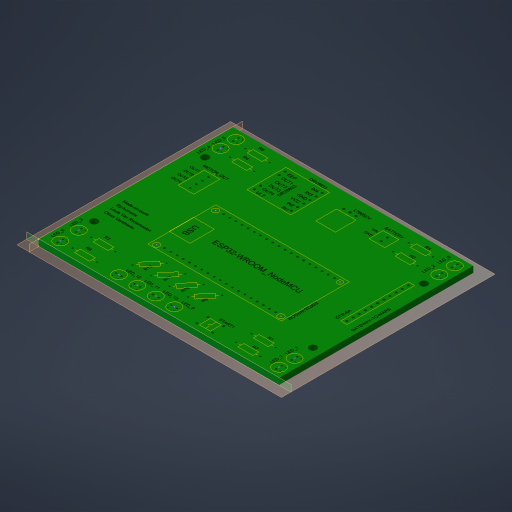
# Autodesk Inventor part: PCB
Saved by Autodesk Inventor 2024 (Build 280153000, 153)
## iProperties
Manager: Louis Van Roosmaelen
Company: DCS - DIGITAL COMBAT SIMULATOR
Created: 2023-12-13
Part Number: PCB
Material: S235
Catalog Web Link: http://emmausbovenbouw.op-weg.be/
Vendor: Emmaüsinstituut Bovenbouw Aalter
Document SubType Name: Modeling
Designer: Louis
Engineer: Declercq St.
Manufacturer: Standard
Standards Organization: Custom
Density: 7.86 g/cm^3
Appearance: Steel
IDENT.NR.: AJ2022
TEAM: 30
Title: F18C Home Cockpit
Author: Louis
Keywords: Ø
Autodesk Inventor part; units mm, degrees
sketch "Outline" plane through (0, 0, 0) normal (0, 0, 1) x (1, 0, 0)
  line L0 (0, 80) -> (99.0602, 80.0102)
  line L1 (99.0602, 80.0102) -> (99.0602, 0)
  line L2 (99.0602, 0) -> (0, 0)
  line L3 (0, 0) -> (0, 80)
  constraints: 8 end point
extrude "Extrusion2" add sketch "Outline" along normal blind 2.5
sketch "Sketch3" plane through (0, 0, 2.5) normal (0, 0, 1) x (1, 0, 0)
  circle A0 centre (71.3201, 72.3901) radius 0.5169
  circle A1 centre (71.32, 72.3901) radius 0.7754
  circle A2 centre (92.7102, 44.4501) radius 0.5159
  circle A3 centre (5.08, 75.0601) radius 0.4226
  circle A4 centre (71.3201, 69.8501) radius 0.5169
  circle A5 centre (71.32, 69.8501) radius 0.7754
  circle A6 centre (5.08, 75.0602) radius 0.9508
  circle A7 centre (92.7102, 44.4501) radius 0.8254
  circle A8 centre (12.9, 57.15) radius 0.4369
  circle A9 centre (12.8999, 57.1499) radius 0.6554
  circle A10 centre (87.5502, 68.5801) radius 0.3637
  circle A11 centre (5.08, 77.3402) radius 0.4226
  circle A12 centre (12.9, 54.61) radius 0.4369
  circle A13 centre (12.8999, 54.6099) radius 0.6554
  circle A14 centre (5.08, 77.3404) radius 0.9508
  circle A15 centre (87.5502, 68.5801) radius 0.6754
  circle A16 centre (12.9, 52.07) radius 0.4369
  circle A17 centre (12.8999, 52.0699) radius 0.6554
  circle A18 centre (92.7102, 41.9101) radius 0.5159
  circle A19 centre (50.93, 3.81) radius 0.4226
  circle A20 centre (12.9, 49.53) radius 0.4369
  circle A21 centre (12.8999, 49.5298) radius 0.6554
  circle A22 centre (50.9301, 3.81) radius 0.9508
  circle A23 centre (92.7102, 41.9101) radius 0.8254
  circle A24 centre (26.6701, 62.2301) radius 0.544
  circle A25 centre (26.6701, 62.2301) radius 0.8
  circle A26 centre (10.24, 68.5801) radius 0.3637
  circle A27 centre (53.2101, 3.81) radius 0.4226
  circle A28 centre (26.6701, 64.7701) radius 0.544
  circle A29 centre (26.6701, 64.7701) radius 0.8
  circle A30 centre (53.2103, 3.81) radius 0.9508
  circle A31 centre (10.24, 68.5801) radius 0.6754
  circle A32 centre (26.6701, 67.3101) radius 0.544
  circle A33 centre (26.6701, 67.3101) radius 0.8
  circle A34 centre (92.7102, 39.3701) radius 0.5159
  circle A35 centre (43.31, 3.81) radius 0.4226
  circle A36 centre (26.6701, 69.8501) radius 0.544
  circle A37 centre (26.6701, 69.8501) radius 0.8
  circle A38 centre (43.3101, 3.81) radius 0.9508
  circle A39 centre (92.7102, 39.3701) radius 0.8254
  circle A40 centre (26.6701, 72.3901) radius 0.544
  circle A41 centre (26.6701, 72.3901) radius 0.8
  circle A42 centre (20.24, 11.43) radius 0.3637
  circle A43 centre (45.5901, 3.81) radius 0.4226
  circle A44 centre (26.6701, 74.9301) radius 0.544
  circle A45 centre (26.6701, 74.9301) radius 0.8
  circle A46 centre (45.5903, 3.81) radius 0.9508
  circle A47 centre (20.24, 11.43) radius 0.6754
  circle A48 centre (41.9101, 62.2301) radius 0.544
  circle A49 centre (41.9101, 62.2301) radius 0.8
  circle A50 centre (92.7102, 36.8301) radius 0.5159
  circle A51 centre (35.69, 3.81) radius 0.4226
  circle A52 centre (41.9101, 64.7701) radius 0.544
  circle A53 centre (41.9101, 64.7701) radius 0.8
  circle A54 centre (35.6901, 3.81) radius 0.9508
  circle A55 centre (92.7102, 36.8301) radius 0.8254
  circle A56 centre (41.9101, 67.3101) radius 0.544
  circle A57 centre (41.9101, 67.3101) radius 0.8
  circle A58 centre (87.5502, 74.9301) radius 0.3637
  circle A59 centre (37.9701, 3.81) radius 0.4226
  circle A60 centre (41.9101, 69.8501) radius 0.544
  circle A61 centre (41.9101, 69.8501) radius 0.8
  circle A62 centre (37.9703, 3.81) radius 0.9508
  circle A63 centre (87.5502, 74.9301) radius 0.6754
  circle A64 centre (41.9101, 72.3901) radius 0.544
  circle A65 centre (41.9101, 72.3901) radius 0.8
  circle A66 centre (92.7102, 34.2901) radius 0.5159
  circle A67 centre (28.07, 3.81) radius 0.4226
  circle A68 centre (41.9101, 74.9301) radius 0.544
  circle A69 centre (41.9101, 74.9301) radius 0.8
  circle A70 centre (28.0701, 3.81) radius 0.9508
  circle A71 centre (92.7102, 34.2901) radius 0.8254
  circle A72 centre (95.2502, 9.0199) radius 0.4226
  circle A73 centre (95.2502, 9.0201) radius 0.9508
  circle A74 centre (10.24, 11.43) radius 0.3637
  circle A75 centre (30.3501, 3.81) radius 0.4226
  circle A76 centre (95.2502, 11.3001) radius 0.4226
  circle A77 centre (95.2502, 11.3002) radius 0.9508
  circle A78 centre (30.3503, 3.81) radius 0.9508
  circle A79 centre (10.24, 11.43) radius 0.6754
  circle A80 centre (95.2502, 68.7101) radius 0.4226
  circle A81 centre (95.2502, 68.7102) radius 0.9508
  circle A82 centre (77.5502, 10.16) radius 0.3637
  circle A83 centre (92.7102, 59.6901) radius 0.5159
  circle A84 centre (95.2502, 70.9902) radius 0.4226
  circle A85 centre (95.2502, 70.9903) radius 0.9508
  circle A86 centre (77.5502, 10.16) radius 0.6754
  circle A87 centre (92.7102, 57.1501) radius 0.5159
  circle A88 centre (5.08, 10.2899) radius 0.4226
  circle A89 centre (5.08, 10.2901) radius 0.9508
  circle A90 centre (92.7102, 57.1501) radius 0.8254
  circle A91 centre (77.5502, 74.9301) radius 0.3637
  circle A92 centre (5.08, 12.5701) radius 0.4226
  circle A93 centre (5.08, 12.5702) radius 0.9508
  circle A94 centre (77.5502, 74.9301) radius 0.6754
  circle A95 centre (92.7102, 54.6101) radius 0.5159
  circle A96 centre (5.08, 68.7101) radius 0.4226
  circle A97 centre (5.08, 68.7102) radius 0.9508
  circle A98 centre (92.7102, 54.6101) radius 0.8254
  circle A99 centre (87.5502, 10.16) radius 0.3637
  circle A100 centre (5.08, 70.9902) radius 0.4226
  circle A101 centre (5.08, 70.9903) radius 0.9508
  circle A102 centre (87.5502, 10.16) radius 0.6754
  circle A103 centre (92.7102, 52.0701) radius 0.5159
  circle A104 centre (95.2502, 75.0601) radius 0.4226
  circle A105 centre (95.2502, 75.0602) radius 0.9508
  circle A106 centre (92.7102, 52.0701) radius 0.8254
  circle A107 centre (20.24, 68.5801) radius 0.3637
  circle A108 centre (95.2502, 77.3402) radius 0.4226
  circle A109 centre (95.2502, 77.3404) radius 0.9508
  circle A110 centre (20.24, 68.5801) radius 0.6754
  circle A111 centre (92.7102, 49.5301) radius 0.5159
  circle A112 centre (5.08, 2.6699) radius 0.4226
  circle A113 centre (5.08, 2.6701) radius 0.9508
  circle A114 centre (92.7102, 49.5301) radius 0.8254
  circle A115 centre (77.5502, 68.5801) radius 0.3637
  circle A116 centre (5.08, 4.95) radius 0.4226
  circle A117 centre (5.08, 4.9502) radius 0.9508
  circle A118 centre (77.5502, 68.5801) radius 0.6754
  circle A119 centre (92.7102, 46.9901) radius 0.5159
  circle A120 centre (95.2502, 2.6699) radius 0.4226
  circle A121 centre (95.2502, 2.6701) radius 0.9508
  circle A122 centre (92.7102, 46.9901) radius 0.8254
  circle A123 centre (20.24, 3.81) radius 0.3637
  circle A124 centre (95.2502, 4.95) radius 0.4226
  circle A125 centre (95.2502, 4.9502) radius 0.9508
  circle A126 centre (20.24, 3.81) radius 0.6754
  circle A127 centre (10.24, 3.81) radius 0.3637
  circle A128 centre (10.24, 3.81) radius 0.6754
  circle A129 centre (77.5502, 3.81) radius 0.3637
  circle A130 centre (77.5502, 3.81) radius 0.6754
  circle A131 centre (87.5502, 3.81) radius 0.3637
  circle A132 centre (87.5502, 3.81) radius 0.6754
  circle A133 centre (20.24, 74.9301) radius 0.3637
  circle A134 centre (20.24, 74.9301) radius 0.6754
  circle A135 centre (10.24, 74.9301) radius 0.3637
  circle A136 centre (10.24, 74.9301) radius 0.6754
  circle A137 centre (57.8241, 17.8003) radius 0.3637
  circle A138 centre (57.824, 17.8004) radius 0.6754
  circle A139 centre (51.3962, 10.1398) radius 0.3637
  circle A140 centre (51.3962, 10.1397) radius 0.6754
  circle A141 centre (50.204, 17.8002) radius 0.3637
  circle A142 centre (50.204, 17.8004) radius 0.6754
  circle A143 centre (43.7762, 10.1398) radius 0.3637
  circle A144 centre (43.7762, 10.1397) radius 0.6754
  circle A145 centre (42.584, 17.8003) radius 0.3637
  circle A146 centre (42.5839, 17.8004) radius 0.6754
  circle A147 centre (36.1561, 10.1398) radius 0.3637
  circle A148 centre (36.1562, 10.1397) radius 0.6754
  circle A149 centre (34.964, 17.8003) radius 0.3637
  circle A150 centre (34.9639, 17.8004) radius 0.6754
  circle A151 centre (28.5361, 10.1398) radius 0.3637
  circle A152 centre (28.5362, 10.1397) radius 0.6754
  circle A153 centre (62.6802, 2.54) radius 0.5167
  circle A154 centre (62.6802, 2.54) radius 0.7874
  circle A155 centre (69.1801, 2.54) radius 0.5167
  circle A156 centre (69.1801, 2.54) radius 0.7874
  circle A157 centre (69.1801, 7.0399) radius 0.5167
  circle A158 centre (69.1801, 7.0399) radius 0.7874
  circle A159 centre (62.6802, 7.0399) radius 0.5167
  circle A160 centre (62.6802, 7.0399) radius 0.7874
  circle A161 centre (52.0701, 73.6601) radius 0.5672
  circle A162 centre (54.6101, 73.6601) radius 0.5672
  circle A163 centre (54.6101, 73.6601) radius 0.825
  circle A164 centre (57.1501, 73.6601) radius 0.5672
  circle A165 centre (57.1501, 73.6601) radius 0.825
  circle A166 centre (74.9301, 22.733) radius 0.4877
  circle A167 centre (74.9301, 22.733) radius 0.8128
  circle A168 centre (72.3901, 22.733) radius 0.4877
  circle A169 centre (72.3901, 22.733) radius 0.8128
  circle A170 centre (69.8501, 22.733) radius 0.4877
  circle A171 centre (69.8501, 22.733) radius 0.8128
  circle A172 centre (67.3101, 22.733) radius 0.4877
  circle A173 centre (67.3101, 22.733) radius 0.8128
  circle A174 centre (64.7701, 22.733) radius 0.4877
  circle A175 centre (64.7701, 22.733) radius 0.8128
  circle A176 centre (62.2301, 22.733) radius 0.4877
  circle A177 centre (62.2301, 22.733) radius 0.8128
  circle A178 centre (59.6901, 22.733) radius 0.4877
  circle A179 centre (59.6901, 22.733) radius 0.8128
  circle A180 centre (57.1501, 22.733) radius 0.4877
  circle A181 centre (57.1501, 22.733) radius 0.8128
  circle A182 centre (54.6101, 22.733) radius 0.4877
  circle A183 centre (54.6101, 22.733) radius 0.8128
  circle A184 centre (52.0701, 22.733) radius 0.4877
  circle A185 centre (52.0701, 22.733) radius 0.8128
  circle A186 centre (49.5301, 22.733) radius 0.4877
  circle A187 centre (49.5301, 22.733) radius 0.8128
  circle A188 centre (46.9901, 22.733) radius 0.4877
  circle A189 centre (46.9901, 22.733) radius 0.8128
  circle A190 centre (44.4501, 22.733) radius 0.4877
  circle A191 centre (44.4501, 22.733) radius 0.8128
  circle A192 centre (41.9101, 22.733) radius 0.4877
  circle A193 centre (41.9101, 22.733) radius 0.8128
  circle A194 centre (39.3701, 22.733) radius 0.4877
  circle A195 centre (39.3701, 22.733) radius 0.8128
  circle A196 centre (36.8301, 22.733) radius 0.4877
  circle A197 centre (36.8301, 22.733) radius 0.8128
  circle A198 centre (34.2901, 22.733) radius 0.4877
  circle A199 centre (34.2901, 22.733) radius 0.8128
  circle A200 centre (31.7501, 22.733) radius 0.4877
  circle A201 centre (31.7501, 22.733) radius 0.8128
  circle A202 centre (29.0831, 22.733) radius 0.4877
  circle A203 centre (29.0831, 22.733) radius 0.8128
  circle A204 centre (29.151, 47.0041) radius 0.4877
  circle A205 centre (29.1509, 47.0041) radius 0.8128
  circle A206 centre (31.691, 47.0041) radius 0.4877
  circle A207 centre (31.6909, 47.0041) radius 0.8128
  circle A208 centre (34.231, 47.0041) radius 0.4877
  circle A209 centre (34.2309, 47.0041) radius 0.8128
  circle A210 centre (36.771, 47.0041) radius 0.4877
  circle A211 centre (36.7709, 47.0041) radius 0.8128
  circle A212 centre (39.311, 47.0041) radius 0.4877
  circle A213 centre (39.3109, 47.0041) radius 0.8128
  circle A214 centre (41.851, 47.0041) radius 0.4877
  circle A215 centre (41.8509, 47.0041) radius 0.8128
  circle A216 centre (44.391, 47.0041) radius 0.4877
  circle A217 centre (44.3909, 47.0041) radius 0.8128
  circle A218 centre (46.931, 47.0041) radius 0.4877
  circle A219 centre (46.9309, 47.0041) radius 0.8128
  circle A220 centre (49.471, 47.0041) radius 0.4877
  circle A221 centre (49.4709, 47.0041) radius 0.8128
  circle A222 centre (52.011, 47.0041) radius 0.4877
  circle A223 centre (52.0109, 47.0041) radius 0.8128
  circle A224 centre (54.5511, 47.0041) radius 0.4877
  circle A225 centre (54.5509, 47.0041) radius 0.8128
  circle A226 centre (57.0911, 47.0041) radius 0.4877
  circle A227 centre (57.0909, 47.0041) radius 0.8128
  circle A228 centre (59.6311, 47.0041) radius 0.4877
  circle A229 centre (59.6309, 47.0041) radius 0.8128
  circle A230 centre (62.1711, 47.0041) radius 0.4877
  circle A231 centre (62.1709, 47.0041) radius 0.8128
  circle A232 centre (64.7111, 47.0041) radius 0.4877
  circle A233 centre (64.7109, 47.0041) radius 0.8128
  circle A234 centre (67.2511, 47.0041) radius 0.4877
  circle A235 centre (67.251, 47.0041) radius 0.8128
  circle A236 centre (69.7911, 47.0041) radius 0.4877
  circle A237 centre (69.791, 47.0041) radius 0.8128
  circle A238 centre (72.3311, 47.0041) radius 0.4877
  circle A239 centre (72.331, 47.0041) radius 0.8128
  circle A240 centre (74.8711, 47.0041) radius 0.4877
  circle A241 centre (74.871, 47.0041) radius 0.8128
  circle A242 centre (50.7028, 49.1306) radius 0.1525
  circle A243 centre (45.1308, 15.6431) radius 0.1525
  circle A244 centre (33.8692, 67.4216) radius 0.1525
  circle A245 centre (37.2901, 36.6408) radius 0.1525
  circle A246 centre (48.8237, 31.0594) radius 0.1525
  circle A247 centre (10.3066, 42.2758) radius 0.1525
  circle A248 centre (46.1262, 42.2758) radius 0.1525
  circle A249 centre (43.7127, 17.5718) radius 0.1525
  circle A250 centre (72.3282, 45.4112) radius 0.1525
  circle A251 centre (87.5502, 74.9301) radius 0.65
  circle A252 centre (20.24, 3.81) radius 0.35
  circle A253 centre (20.24, 3.81) radius 0.65
  circle A254 centre (71.3201, 72.3901) radius 0.5
  circle A255 centre (71.32, 72.3901) radius 0.75
  circle A256 centre (10.24, 3.81) radius 0.35
  circle A257 centre (10.24, 3.81) radius 0.65
  circle A258 centre (71.3201, 69.8501) radius 0.5
  circle A259 centre (71.32, 69.8501) radius 0.75
  circle A260 centre (77.5502, 3.81) radius 0.35
  circle A261 centre (77.5502, 3.81) radius 0.65
  circle A262 centre (12.9, 57.15) radius 0.42
  circle A263 centre (12.8999, 57.1499) radius 0.63
  circle A264 centre (87.5502, 3.81) radius 0.35
  circle A265 centre (87.5502, 3.81) radius 0.65
  circle A266 centre (12.9, 54.61) radius 0.42
  circle A267 centre (12.8999, 54.6099) radius 0.63
  circle A268 centre (20.24, 74.9301) radius 0.35
  circle A269 centre (20.24, 74.9301) radius 0.65
  circle A270 centre (12.9, 52.07) radius 0.42
  circle A271 centre (12.8999, 52.0699) radius 0.63
  circle A272 centre (10.24, 74.9301) radius 0.35
  circle A273 centre (10.24, 74.9301) radius 0.65
  circle A274 centre (12.9, 49.53) radius 0.42
  circle A275 centre (12.8999, 49.5298) radius 0.63
  circle A276 centre (57.8241, 17.8003) radius 0.35
  circle A277 centre (57.824, 17.8004) radius 0.65
  circle A278 centre (26.6701, 62.2301) radius 0.51
  circle A279 centre (26.6701, 62.2301) radius 0.75
  circle A280 centre (51.3962, 10.1398) radius 0.35
  circle A281 centre (51.3962, 10.1397) radius 0.65
  circle A282 centre (26.6701, 64.7701) radius 0.51
  circle A283 centre (26.6701, 64.7701) radius 0.75
  circle A284 centre (50.204, 17.8002) radius 0.35
  circle A285 centre (50.204, 17.8004) radius 0.65
  circle A286 centre (26.6701, 67.3101) radius 0.51
  circle A287 centre (26.6701, 67.3101) radius 0.75
  circle A288 centre (43.7762, 10.1398) radius 0.35
  circle A289 centre (43.7762, 10.1397) radius 0.65
  circle A290 centre (26.6701, 69.8501) radius 0.51
  circle A291 centre (26.6701, 69.8501) radius 0.75
  circle A292 centre (42.584, 17.8003) radius 0.35
  circle A293 centre (42.5839, 17.8004) radius 0.65
  circle A294 centre (26.6701, 72.3901) radius 0.51
  circle A295 centre (26.6701, 72.3901) radius 0.75
  circle A296 centre (36.1561, 10.1398) radius 0.35
  circle A297 centre (36.1562, 10.1397) radius 0.65
  circle A298 centre (26.6701, 74.9301) radius 0.51
  circle A299 centre (26.6701, 74.9301) radius 0.75
  circle A300 centre (34.964, 17.8003) radius 0.35
  circle A301 centre (34.9639, 17.8004) radius 0.65
  circle A302 centre (41.9101, 62.2301) radius 0.51
  circle A303 centre (41.9101, 62.2301) radius 0.75
  circle A304 centre (28.5361, 10.1398) radius 0.35
  circle A305 centre (28.5362, 10.1397) radius 0.65
  circle A306 centre (41.9101, 64.7701) radius 0.51
  circle A307 centre (41.9101, 64.7701) radius 0.75
  circle A308 centre (62.6802, 2.54) radius 0.5
  circle A309 centre (62.6802, 2.54) radius 0.762
  circle A310 centre (41.9101, 67.3101) radius 0.51
  circle A311 centre (41.9101, 67.3101) radius 0.75
  circle A312 centre (69.1801, 2.54) radius 0.5
  circle A313 centre (69.1801, 2.54) radius 0.762
  circle A314 centre (41.9101, 69.8501) radius 0.51
  circle A315 centre (41.9101, 69.8501) radius 0.75
  circle A316 centre (69.1801, 7.0399) radius 0.5
  circle A317 centre (69.1801, 7.0399) radius 0.762
  circle A318 centre (41.9101, 72.3901) radius 0.51
  circle A319 centre (41.9101, 72.3901) radius 0.75
  circle A320 centre (62.6802, 7.0399) radius 0.5
  circle A321 centre (62.6802, 7.0399) radius 0.762
  circle A322 centre (41.9101, 74.9301) radius 0.51
  circle A323 centre (52.0701, 73.6601) radius 0.55
  circle A324 centre (41.9101, 74.9301) radius 0.75
  circle A325 centre (95.2502, 9.0199) radius 0.4
  circle A326 centre (54.6101, 73.6601) radius 0.55
  circle A327 centre (54.6101, 73.6601) radius 0.8
  circle A328 centre (95.2502, 9.0201) radius 0.9
  circle A329 centre (95.2502, 11.3001) radius 0.4
  circle A330 centre (57.1501, 73.6601) radius 0.55
  circle A331 centre (57.1501, 73.6601) radius 0.8
  circle A332 centre (95.2502, 11.3002) radius 0.9
  circle A333 centre (95.2502, 68.7101) radius 0.4
  circle A334 centre (74.9301, 22.733) radius 0.4572
  circle A335 centre (74.9301, 22.733) radius 0.762
  circle A336 centre (95.2502, 68.7102) radius 0.9
  circle A337 centre (95.2502, 70.9902) radius 0.4
  circle A338 centre (72.3901, 22.733) radius 0.4572
  circle A339 centre (72.3901, 22.733) radius 0.762
  circle A340 centre (95.2502, 70.9903) radius 0.9
  circle A341 centre (5.08, 10.2899) radius 0.4
  circle A342 centre (69.8501, 22.733) radius 0.4572
  circle A343 centre (69.8501, 22.733) radius 0.762
  circle A344 centre (5.08, 10.2901) radius 0.9
  circle A345 centre (5.08, 12.5701) radius 0.4
  circle A346 centre (67.3101, 22.733) radius 0.4572
  circle A347 centre (67.3101, 22.733) radius 0.762
  circle A348 centre (5.08, 12.5702) radius 0.9
  circle A349 centre (5.08, 68.7101) radius 0.4
  circle A350 centre (64.7701, 22.733) radius 0.4572
  circle A351 centre (64.7701, 22.733) radius 0.762
  circle A352 centre (5.08, 68.7102) radius 0.9
  circle A353 centre (5.08, 70.9902) radius 0.4
  circle A354 centre (62.2301, 22.733) radius 0.4572
  circle A355 centre (62.2301, 22.733) radius 0.762
  circle A356 centre (5.08, 70.9903) radius 0.9
  circle A357 centre (95.2502, 75.0601) radius 0.4
  circle A358 centre (59.6901, 22.733) radius 0.4572
  circle A359 centre (59.6901, 22.733) radius 0.762
  circle A360 centre (95.2502, 75.0602) radius 0.9
  circle A361 centre (95.2502, 77.3402) radius 0.4
  circle A362 centre (57.1501, 22.733) radius 0.4572
  circle A363 centre (57.1501, 22.733) radius 0.762
  circle A364 centre (95.2502, 77.3404) radius 0.9
  circle A365 centre (5.08, 2.6699) radius 0.4
  circle A366 centre (54.6101, 22.733) radius 0.4572
  circle A367 centre (54.6101, 22.733) radius 0.762
  circle A368 centre (5.08, 2.6701) radius 0.9
  circle A369 centre (5.08, 4.95) radius 0.4
  circle A370 centre (52.0701, 22.733) radius 0.4572
  circle A371 centre (52.0701, 22.733) radius 0.762
  circle A372 centre (5.08, 4.9502) radius 0.9
  circle A373 centre (95.2502, 2.6699) radius 0.4
  circle A374 centre (49.5301, 22.733) radius 0.4572
  circle A375 centre (49.5301, 22.733) radius 0.762
  circle A376 centre (95.2502, 2.6701) radius 0.9
  circle A377 centre (95.2502, 4.95) radius 0.4
  circle A378 centre (46.9901, 22.733) radius 0.4572
  circle A379 centre (46.9901, 22.733) radius 0.762
  circle A380 centre (95.2502, 4.9502) radius 0.9
  circle A381 centre (5.08, 75.0601) radius 0.4
  circle A382 centre (44.4501, 22.733) radius 0.4572
  circle A383 centre (44.4501, 22.733) radius 0.762
  circle A384 centre (5.08, 75.0602) radius 0.9
  circle A385 centre (5.08, 77.3402) radius 0.4
  circle A386 centre (41.9101, 22.733) radius 0.4572
  circle A387 centre (41.9101, 22.733) radius 0.762
  circle A388 centre (5.08, 77.3404) radius 0.9
  circle A389 centre (50.93, 3.81) radius 0.4
  circle A390 centre (39.3701, 22.733) radius 0.4572
  circle A391 centre (39.3701, 22.733) radius 0.762
  circle A392 centre (50.9301, 3.81) radius 0.9
  circle A393 centre (53.2101, 3.81) radius 0.4
  circle A394 centre (36.8301, 22.733) radius 0.4572
  circle A395 centre (36.8301, 22.733) radius 0.762
  circle A396 centre (53.2103, 3.81) radius 0.9
  circle A397 centre (43.31, 3.81) radius 0.4
  circle A398 centre (34.2901, 22.733) radius 0.4572
  circle A399 centre (34.2901, 22.733) radius 0.762
  circle A400 centre (43.3101, 3.81) radius 0.9
  circle A401 centre (45.5901, 3.81) radius 0.4
  circle A402 centre (31.7501, 22.733) radius 0.4572
  circle A403 centre (31.7501, 22.733) radius 0.762
  circle A404 centre (45.5903, 3.81) radius 0.9
  circle A405 centre (35.69, 3.81) radius 0.4
  circle A406 centre (29.0831, 22.733) radius 0.4572
  circle A407 centre (29.0831, 22.733) radius 0.762
  circle A408 centre (35.6901, 3.81) radius 0.9
  circle A409 centre (37.9701, 3.81) radius 0.4
  circle A410 centre (29.151, 47.0041) radius 0.4572
  circle A411 centre (29.1509, 47.0041) radius 0.762
  circle A412 centre (37.9703, 3.81) radius 0.9
  circle A413 centre (28.07, 3.81) radius 0.4
  circle A414 centre (31.691, 47.0041) radius 0.4572
  circle A415 centre (31.6909, 47.0041) radius 0.762
  circle A416 centre (28.0701, 3.81) radius 0.9
  circle A417 centre (30.3501, 3.81) radius 0.4
  circle A418 centre (34.231, 47.0041) radius 0.4572
  circle A419 centre (34.2309, 47.0041) radius 0.762
  circle A420 centre (30.3503, 3.81) radius 0.9
  circle A421 centre (92.7102, 59.6901) radius 0.5
  circle A422 centre (36.771, 47.0041) radius 0.4572
  circle A423 centre (36.7709, 47.0041) radius 0.762
  circle A424 centre (92.7102, 57.1501) radius 0.5
  circle A425 centre (92.7102, 57.1501) radius 0.8
  circle A426 centre (39.311, 47.0041) radius 0.4572
  circle A427 centre (39.3109, 47.0041) radius 0.762
  circle A428 centre (92.7102, 54.6101) radius 0.5
  circle A429 centre (92.7102, 54.6101) radius 0.8
  circle A430 centre (41.851, 47.0041) radius 0.4572
  circle A431 centre (41.8509, 47.0041) radius 0.762
  circle A432 centre (92.7102, 52.0701) radius 0.5
  circle A433 centre (92.7102, 52.0701) radius 0.8
  circle A434 centre (44.391, 47.0041) radius 0.4572
  circle A435 centre (44.3909, 47.0041) radius 0.762
  circle A436 centre (92.7102, 49.5301) radius 0.5
  circle A437 centre (92.7102, 49.5301) radius 0.8
  circle A438 centre (46.931, 47.0041) radius 0.4572
  circle A439 centre (46.9309, 47.0041) radius 0.762
  circle A440 centre (92.7102, 46.9901) radius 0.5
  circle A441 centre (92.7102, 46.9901) radius 0.8
  circle A442 centre (49.471, 47.0041) radius 0.4572
  circle A443 centre (49.4709, 47.0041) radius 0.762
  circle A444 centre (92.7102, 44.4501) radius 0.5
  circle A445 centre (92.7102, 44.4501) radius 0.8
  circle A446 centre (52.011, 47.0041) radius 0.4572
  circle A447 centre (52.0109, 47.0041) radius 0.762
  circle A448 centre (92.7102, 41.9101) radius 0.5
  circle A449 centre (92.7102, 41.9101) radius 0.8
  circle A450 centre (54.5511, 47.0041) radius 0.4572
  circle A451 centre (54.5509, 47.0041) radius 0.762
  circle A452 centre (92.7102, 39.3701) radius 0.5
  circle A453 centre (92.7102, 39.3701) radius 0.8
  circle A454 centre (57.0911, 47.0041) radius 0.4572
  circle A455 centre (57.0909, 47.0041) radius 0.762
  circle A456 centre (92.7102, 36.8301) radius 0.5
  circle A457 centre (92.7102, 36.8301) radius 0.8
  circle A458 centre (59.6311, 47.0041) radius 0.4572
  circle A459 centre (59.6309, 47.0041) radius 0.762
  circle A460 centre (92.7102, 34.2901) radius 0.5
  circle A461 centre (92.7102, 34.2901) radius 0.8
  circle A462 centre (62.1711, 47.0041) radius 0.4572
  circle A463 centre (62.1709, 47.0041) radius 0.762
  circle A464 centre (77.5502, 10.16) radius 0.35
  circle A465 centre (77.5502, 10.16) radius 0.65
  circle A466 centre (64.7111, 47.0041) radius 0.4572
  circle A467 centre (64.7109, 47.0041) radius 0.762
  circle A468 centre (87.5502, 10.16) radius 0.35
  circle A469 centre (87.5502, 10.16) radius 0.65
  circle A470 centre (67.2511, 47.0041) radius 0.4572
  circle A471 centre (67.251, 47.0041) radius 0.762
  circle A472 centre (77.5502, 68.5801) radius 0.35
  circle A473 centre (77.5502, 68.5801) radius 0.65
  circle A474 centre (69.7911, 47.0041) radius 0.4572
  circle A475 centre (69.791, 47.0041) radius 0.762
  circle A476 centre (87.5502, 68.5801) radius 0.35
  circle A477 centre (87.5502, 68.5801) radius 0.65
  circle A478 centre (72.3311, 47.0041) radius 0.4572
  circle A479 centre (72.331, 47.0041) radius 0.762
  circle A480 centre (20.24, 11.43) radius 0.35
  circle A481 centre (20.24, 11.43) radius 0.65
  circle A482 centre (74.8711, 47.0041) radius 0.4572
  circle A483 centre (74.871, 47.0041) radius 0.762
  circle A484 centre (50.7028, 49.1306) radius 0.305
  circle A485 centre (10.24, 11.43) radius 0.35
  circle A486 centre (45.1308, 15.6431) radius 0.305
  circle A487 centre (10.24, 11.43) radius 0.65
  circle A488 centre (33.8692, 67.4216) radius 0.305
  circle A489 centre (20.24, 68.5801) radius 0.35
  circle A490 centre (37.2901, 36.6408) radius 0.305
  circle A491 centre (20.24, 68.5801) radius 0.65
  circle A492 centre (48.8237, 31.0594) radius 0.305
  circle A493 centre (10.24, 68.5801) radius 0.35
  circle A494 centre (10.3066, 42.2758) radius 0.305
  circle A495 centre (10.24, 68.5801) radius 0.65
  circle A496 centre (46.1262, 42.2758) radius 0.305
  circle A497 centre (77.5502, 74.9301) radius 0.35
  circle A498 centre (43.7127, 17.5718) radius 0.305
  circle A499 centre (77.5502, 74.9301) radius 0.65
  circle A500 centre (72.3282, 45.4112) radius 0.305
  circle A501 centre (87.5502, 74.9301) radius 0.35
  circle A502 centre (95.2502, 63.5001) radius 1.55
  circle A503 centre (5.08, 63.5001) radius 1.55
  circle A504 centre (5.08, 17.78) radius 1.55
  circle A505 centre (95.2502, 17.78) radius 1.55
  point P0 (0, 0)
  constraints: 506 centre point
extrude "Extrusion3" cut sketch "Sketch3" against normal up to surface (2.5 mm away) contours A2 | A10 | A12 | A17 | A28 | A32 | A35 | A36 | A42 | A74 | A80 | A84 | A87 | A104 | A107 | A115 | A119 | A123 | A127 | A141 | A194 | A224 | A230 | A252 | A254 | A256 | A258 | A260 | A262 | A264 | A266 | A268 | A270 | A272 | A274 | A276 | A278 | A280 | A282 | A284 | A288 | A292 | A294 | A296 | A298 | A300 | A302 | A304 | A306 | A308 | A310 | A312 | A314 | A316 | A318 | A320 | A322 | A323 | A325 | A326 | A329 | A330 | A333 | A334 | A337 | A338 | A341 | A342 | A345 | A346 | A349 | A350 | A353 | A354 | A357 | A358 | A361 | A362 | A365 | A366 | A369 | A370 | A373 | A374 | A377 | A378 | A381 | A382 | A385 | A386 | A389 | A390 | A393 | A394 | A397 | A398 | A401 | A402 | A405 | A406 | A409 | A410 | A413 | A414 | A417 | A418 | A421 | A422 | A424 | A426 | A428 | A430 | A432 | A434 | A436 | A438 | A440 | A442 | A444 | A446 | A448 | A450 | A452 | A454 | A456 | A458 | A460 | A462 | A464 | A466 | A468 | A470 | A472 | A474 | A476 | A478 | A480 | A482 | A485 | A489 | A493 | A497 | A501
hole "Hole1" at (5.08, 63.5001, 2.5) at (5.08, 17.78, 2.5) at (95.2502, 63.5001, 2.5) at (95.2502, 17.78, 2.5) direction (0, 0, -1) diameter 3.1 end through all
sketch "Sketch4" plane through (0, 0, 2.5) normal (0, 0, 1) x (1, 0, 0)
  line L0 (67.894, 68.2489) -> (74.3464, 68.2489)
  line L1 (74.3464, 68.2489) -> (74.3464, 73.9913)
  line L2 (74.3464, 73.9913) -> (67.894, 73.9913)
  line L3 (67.894, 73.9913) -> (67.894, 68.2489)
  line L4 (15.9262, 58.7262) -> (15.9262, 47.9538)
  line L5 (15.9262, 47.9538) -> (9.4738, 47.9538)
  line L6 (9.4738, 47.9538) -> (9.4738, 58.7262)
  line L7 (9.4738, 58.7262) -> (15.9262, 58.7262)
  line L8 (25.2911, 76.5801) -> (43.2911, 76.5801)
  line L9 (43.2911, 76.5801) -> (43.2911, 60.5801)
  line L10 (43.2911, 60.5801) -> (25.2911, 60.5801)
  line L11 (25.2911, 60.5801) -> (25.2911, 76.5801)
  line L12 (91.4402, 33.0201) -> (91.4402, 60.9601)
  line L13 (93.9802, 60.9601) -> (93.9802, 33.0201)
  line L14 (93.9306, 33.0391) -> (91.4897, 33.0391)
  line L15 (91.4402, 60.9601) -> (93.8801, 60.9601)
  line L16 (79.474, 10.1635) -> (78.4862, 10.1635)
  line L17 (85.6264, 10.1565) -> (86.6142, 10.1565)
  line L18 (79.474, 11.3862) -> (85.6264, 11.3862)
  line L19 (85.6264, 11.3862) -> (85.6264, 8.9338)
  line L20 (85.6264, 8.9338) -> (79.474, 8.9338)
  line L21 (79.474, 8.9338) -> (79.474, 11.3862)
  line L22 (79.474, 68.5836) -> (78.4862, 68.5836)
  line L23 (85.6264, 68.5767) -> (86.6142, 68.5767)
  line L24 (79.474, 69.8063) -> (85.6264, 69.8063)
  line L25 (85.6264, 69.8063) -> (85.6264, 67.3539)
  line L26 (85.6264, 67.3539) -> (79.474, 67.3539)
  line L27 (79.474, 67.3539) -> (79.474, 69.8063)
  line L28 (18.3162, 11.4265) -> (19.304, 11.4265)
  line L29 (12.1638, 11.4335) -> (11.176, 11.4335)
  line L30 (18.3162, 10.2038) -> (12.1638, 10.2038)
  line L31 (12.1638, 10.2038) -> (12.1638, 12.6562)
  line L32 (12.1638, 12.6562) -> (18.3162, 12.6562)
  line L33 (18.3162, 12.6562) -> (18.3162, 10.2038)
  line L34 (18.3162, 68.5767) -> (19.304, 68.5767)
  line L35 (12.1638, 68.5836) -> (11.176, 68.5836)
  line L36 (18.3162, 67.3539) -> (12.1638, 67.3539)
  line L37 (12.1638, 67.3539) -> (12.1638, 69.8063)
  line L38 (12.1638, 69.8063) -> (18.3162, 69.8063)
  line L39 (18.3162, 69.8063) -> (18.3162, 67.3539)
  line L40 (79.474, 74.9336) -> (78.4862, 74.9336)
  line L41 (85.6264, 74.9267) -> (86.6142, 74.9267)
  line L42 (79.474, 76.1563) -> (85.6264, 76.1563)
  line L43 (85.6264, 76.1563) -> (85.6264, 73.704)
  line L44 (85.6264, 73.704) -> (79.474, 73.704)
  line L45 (79.474, 73.704) -> (79.474, 76.1563)
  line L46 (18.3162, 3.8065) -> (19.304, 3.8065)
  line L47 (12.1638, 3.8135) -> (11.176, 3.8135)
  line L48 (18.3162, 2.5838) -> (12.1638, 2.5838)
  line L49 (12.1638, 2.5838) -> (12.1638, 5.0362)
  line L50 (12.1638, 5.0362) -> (18.3162, 5.0362)
  line L51 (18.3162, 5.0362) -> (18.3162, 2.5838)
  line L52 (79.474, 3.8135) -> (78.4862, 3.8135)
  line L53 (85.6264, 3.8065) -> (86.6142, 3.8065)
  line L54 (79.474, 5.0362) -> (85.6264, 5.0362)
  line L55 (85.6264, 5.0362) -> (85.6264, 2.5838)
  line L56 (85.6264, 2.5838) -> (79.474, 2.5838)
  line L57 (79.474, 2.5838) -> (79.474, 5.0362)
  line L58 (18.3162, 74.9267) -> (19.304, 74.9267)
  line L59 (12.1638, 74.9336) -> (11.176, 74.9336)
  line L60 (18.3162, 73.704) -> (12.1638, 73.704)
  line L61 (12.1638, 73.704) -> (12.1638, 76.1563)
  line L62 (12.1638, 76.1563) -> (18.3162, 76.1563)
  line L63 (18.3162, 76.1563) -> (18.3162, 73.704)
  line L64 (56.5901, 16.3243) -> (57.2251, 17.081)
  line L65 (52.6301, 11.6157) -> (51.9951, 10.8591)
  line L66 (57.5268, 15.5384) -> (53.5721, 10.8253)
  line L67 (53.5721, 10.8253) -> (51.6934, 12.4017)
  line L68 (51.6934, 12.4017) -> (55.6481, 17.1147)
  line L69 (55.6481, 17.1147) -> (57.5268, 15.5384)
  line L70 (48.9701, 16.3243) -> (49.6051, 17.081)
  line L71 (45.0101, 11.6157) -> (44.3751, 10.8591)
  line L72 (49.9067, 15.5384) -> (45.9521, 10.8253)
  line L73 (45.9521, 10.8253) -> (44.0735, 12.4017)
  line L74 (44.0735, 12.4017) -> (48.0281, 17.1147)
  line L75 (48.0281, 17.1147) -> (49.9067, 15.5384)
  line L76 (41.3501, 16.3243) -> (41.985, 17.081)
  line L77 (37.3901, 11.6157) -> (36.7551, 10.8591)
  line L78 (42.2867, 15.5384) -> (38.3321, 10.8253)
  line L79 (38.3321, 10.8253) -> (36.4534, 12.4017)
  line L80 (36.4534, 12.4017) -> (40.4081, 17.1147)
  line L81 (40.4081, 17.1147) -> (42.2867, 15.5384)
  line L82 (33.7301, 16.3243) -> (34.365, 17.081)
  line L83 (29.7701, 11.6157) -> (29.1351, 10.8591)
  line L84 (34.6667, 15.5384) -> (30.712, 10.8253)
  line L85 (30.712, 10.8253) -> (28.8334, 12.4017)
  line L86 (28.8334, 12.4017) -> (32.7881, 17.1147)
  line L87 (32.7881, 17.1147) -> (34.6667, 15.5384)
  line L88 (63.6801, 2.54) -> (68.1801, 2.54)
  line L89 (68.1801, 2.54) -> (68.1801, 7.04)
  line L90 (68.1801, 7.04) -> (63.6801, 7.04)
  line L91 (63.6801, 7.04) -> (63.6801, 2.54)
  line L92 (66.1798, 7.0409) -> (66.1798, 5.5398)
  line L93 (66.1798, 5.5398) -> (65.1801, 4.54)
  line L94 (66.1801, 3.54) -> (66.1801, 2.54)
  line L95 (66.1801, 3.54) -> (66.1801, 3.04)
  line L96 (66.1801, 4.04) -> (66.1801, 2.54)
  line L97 (58.6201, 72.0301) -> (58.6201, 63.6101)
  line L98 (58.6201, 63.6101) -> (50.6001, 63.6101)
  line L99 (50.6001, 63.6101) -> (50.6001, 72.1601)
  line L100 (58.6201, 72.0301) -> (58.6201, 72.1601)
  line L101 (50.6601, 72.1601) -> (58.5601, 72.1601)
  line L102 (57.1501, 72.479) -> (57.1501, 72.1601)
  line L103 (54.6101, 72.479) -> (54.6101, 72.1601)
  line L104 (52.0701, 72.1601) -> (52.0701, 72.479)
  line L105 (32.6434, 39.7176) -> (32.6434, 29.6845)
  line L106 (32.6434, 29.6845) -> (24.1344, 29.6845)
  line L107 (24.1344, 29.6845) -> (24.1344, 39.7176)
  line L108 (24.1344, 39.7176) -> (32.6434, 39.7176)
  line L109 (79.2482, 48.7681) -> (79.2482, 20.7681)
  line L110 (79.2482, 20.7681) -> (24.2482, 20.7681)
  line L111 (24.2482, 20.7681) -> (24.2482, 48.7681)
  line L112 (24.2482, 48.7681) -> (79.2482, 48.7681)
  circle A0 centre (12.8999, 59.4361) radius 0.08
  circle A1 centre (95.2502, 10.1631) radius 2.5001
  circle A2 centre (95.2502, 69.8532) radius 2.5001
  circle A3 centre (5.08, 11.4331) radius 2.5001
  circle A4 centre (5.08, 69.8532) radius 2.5001
  circle A5 centre (95.2502, 76.2032) radius 2.5001
  circle A6 centre (5.08, 3.8131) radius 2.5001
  circle A7 centre (95.2502, 3.8131) radius 2.5001
  circle A8 centre (5.08, 76.2032) radius 2.5001
  circle A9 centre (52.0732, 3.81) radius 2.5001
  circle A10 centre (44.4531, 3.81) radius 2.5001
  circle A11 centre (36.8331, 3.81) radius 2.5001
  circle A12 centre (29.2131, 3.81) radius 2.5001
  circle A13 centre (26.3569, 22.255) radius 1.2499
  circle A14 centre (77.411, 22.382) radius 1.2499
  circle A15 centre (77.411, 46.7661) radius 1.125
  circle A16 centre (26.2299, 46.6391) radius 1.2499
  point P0 (0, 0)
  point P1 (3.81, 22.86)
  point P2 (3.81, 27.9401)
  point P3 (3.81, 30.4801)
  point P4 (3.81, 25.4001)
  point P5 (97.7902, 31.7501)
  point P6 (67.3101, 74.9301)
  point P7 (65.0241, 71.8821)
  point P8 (64.5161, 69.3421)
  point P9 (7.62, 59.6901)
  point P10 (5.334, 56.6421)
  point P11 (5.334, 54.1021)
  point P12 (5.334, 51.5621)
  point P13 (5.334, 49.0221)
  point P14 (34.2911, 76.8352)
  point P15 (38.6441, 61.143)
  point P16 (38.1539, 63.683)
  point P17 (37.1709, 66.223)
  point P18 (37.336, 68.763)
  point P19 (38.1539, 71.303)
  point P20 (38.1006, 73.843)
  point P21 (28.0676, 61.143)
  point P22 (28.0676, 63.683)
  point P23 (28.1946, 66.223)
  point P24 (28.1946, 68.763)
  point P25 (28.1946, 71.303)
  point P26 (28.1946, 73.843)
  point P27 (34.4359, 64.7767)
  point P28 (92.4562, 10.0231)
  point P29 (97.0282, 8.8931)
  point P30 (97.0282, 11.1791)
  point P31 (91.4402, 67.3101)
  point P32 (97.0282, 68.5832)
  point P33 (97.0282, 70.8692)
  point P34 (2.286, 11.2931)
  point P35 (6.858, 10.1631)
  point P36 (6.858, 12.4491)
  point P37 (2.54, 63.5001)
  point P38 (6.858, 68.5832)
  point P39 (6.858, 70.8692)
  point P40 (91.4402, 73.6601)
  point P41 (97.0282, 74.9332)
  point P42 (97.0282, 77.2192)
  point P43 (2.286, 3.6731)
  point P44 (6.858, 2.5431)
  point P45 (6.858, 4.8291)
  point P46 (92.4562, 3.6731)
  point P47 (97.0282, 2.5431)
  point P48 (97.0282, 4.8291)
  point P49 (2.54, 69.8501)
  point P50 (6.858, 74.9332)
  point P51 (6.858, 77.2192)
  point P52 (51.9332, 6.604)
  point P53 (50.8031, 2.032)
  point P54 (53.0892, 2.032)
  point P55 (44.3132, 6.604)
  point P56 (43.1831, 2.032)
  point P57 (45.4691, 2.032)
  point P58 (36.6932, 6.604)
  point P59 (35.5631, 2.032)
  point P60 (37.8491, 2.032)
  point P61 (29.0732, 6.604)
  point P62 (27.9431, 2.032)
  point P63 (30.2291, 2.032)
  point P64 (90.1702, 33.0201)
  point P65 (82.2962, 11.684)
  point P66 (82.2962, 70.1041)
  point P67 (12.7, 13.97)
  point P68 (12.7, 71.1201)
  point P69 (82.2962, 76.4542)
  point P70 (12.7, 6.35)
  point P71 (82.2962, 5.334)
  point P72 (12.7, 77.4702)
  point P73 (56.5321, 11.4199)
  point P74 (48.6881, 10.7925)
  point P75 (41.1539, 11.0871)
  point P76 (33.3366, 10.8039)
  point P77 (65.7861, 8.128)
  point P78 (54.6101, 74.9301)
  point P79 (79.5022, 34.7981)
  point P80 (27.1189, 37.368)
  point P81 (36.8301, 34.2901)
  constraints: 226 end point, 17 centre point, 81 other
body "Solid2"
